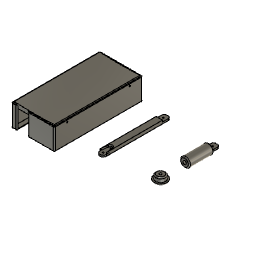
WP_Switch v2 (Autodesk Fusion 360 design; units mm, degrees)
Autodesk Fusion 360 part; units mm, degrees
sketch "Skizze1" plane through (0, 0, 0) normal (0, 1, 0) x (1, 0, 0)
  line L0 (18.75, -0.5552) -> (18.75, 3.444)
  line L1 (18.75, 3.444) -> (-18.75, 3.444)
  line L2 (-18.75, 3.444) -> (-18.75, -0.556)
  arc A0 (18.75, -0.5552) -> (-18.75, -0.556) centre (0.0063, -299.9691) ccw
  dimension "d1" = 600
  dimension "d2" = 37.5
  dimension "d3" = 18.75
  dimension "d4" = 4
  constraint vertical L0
  constraint horizontal L1
  constraint vertical L2
  measures "d1" diameter of A0
  measures "d2" distance of L2.end L0.start
  measures "d3" horizontal distance of origin L2.end
  measures "d4" distance of L2.end L1.end
extrude "Extrusion2" add sketch "Skizze1" along normal blind 80 makes body 1
sketch "Skizze2" plane through (0, 0, -3.444) normal (0, 0, -1) x (1, 0, 0)
  line L0 (18.75, 0) -> (-18.75, 0)
  line L1 (-18.75, 0) -> (-18.75, -80)
  line L2 (-18.75, -80) -> (18.75, -80)
  line L3 (18.75, -80) -> (18.75, 0)
  line L4 (-18.75, 0) -> (18.75, -80) construction
  line L5 (18.75, 0) -> (-18.75, -80) construction
  line L6 (19, 0.25) -> (-19, 0.25)
  line L7 (-19, 0.25) -> (-19, -80.25)
  line L8 (-19, -80.25) -> (19, -80.25)
  line L9 (19, -80.25) -> (19, 0.25)
  line L10 (19, 0.25) -> (-19, -80.25) construction
  line L11 (-19, 0.25) -> (19, -80.25) construction
  line L12 (-20, -81.25) -> (20, -81.25)
  line L13 (20, -81.25) -> (20, 1.25)
  line L14 (20, 1.25) -> (-20, 1.25)
  line L15 (-20, 1.25) -> (-20, -81.25)
  point P0 (0, -40)
  dimension "d9" = 38
  dimension "d10" = 80.5
  dimension "d11" = 1
  constraint coincident L0.end L1.start
  constraint coincident L2.end L3.start
  constraint coincident L0.start L3.end
  constraint coincident L1.end L2.start
  constraint horizontal L6
  constraint perpendicular L6 L7
  constraint parallel L6 L8
  constraint parallel L7 L9
  constraint coincident L10 P0
  constraint coincident L11 P0
  constraint midpoint L5 P0
  measures "d9" distance of L7.end L8.end
  measures "d10" distance of L6.end L7.end
extrude "Extrusion3" add sketch "Skizze2" along normal blind 16 and the other way blind 3 separate body contours L12 L13 L14 L15 makes body 2
sketch "Skizze3" plane through (0, 0, -3.444) normal (0, 0, -1) x (1, 0, 0)
  line L0 (18.75, 0) -> (-18.75, 0)
  line L1 (-18.75, 0) -> (-18.75, -80)
  line L2 (-18.75, -80) -> (18.75, -80)
  line L3 (18.75, -80) -> (18.75, 0)
  line L4 (-1, -3.1253) -> (6, -3.1253)
  line L5 (6, -3.1253) -> (6, -8.3753)
  line L6 (6, -8.3753) -> (-1, -8.3753)
  line L7 (-1, -8.3753) -> (-1, -3.1253)
  line L8 (-1, -28.3753) -> (6, -28.3753)
  line L9 (6, -28.3753) -> (6, -33.6253)
  line L10 (6, -33.6253) -> (-1, -33.6253)
  line L11 (-1, -33.6253) -> (-1, -28.3753)
  line L12 (-1, -8.3753) -> (-1, -28.3753) construction
  line L13 (-18.75, 0) -> (18.75, -80) construction
  line L14 (18.75, 0) -> (-18.75, -80) construction
  line L15 (-16.9509, -3.8381) -> (16.9509, -3.8381)
  line L16 (16.9509, -3.8381) -> (16.9509, -33.6785)
  line L17 (16.9509, -33.6785) -> (-16.9509, -33.6785)
  line L18 (-16.9509, -33.6785) -> (-16.9509, -3.8381)
  dimension "d16" = 7
  dimension "d17" = 5.25
  dimension "d18" = 7
  dimension "d19" = 5.25
  dimension "d20" = 20
  dimension "d23" = 1
  constraint horizontal L4
  constraint vertical L5
  constraint horizontal L6
  constraint vertical L7
  constraint horizontal L8
  constraint vertical L9
  constraint horizontal L10
  constraint vertical L11
  constraint perpendicular L8 L12
  constraint coincident L0.end L1.start
  constraint coincident L2.end L3.start
  constraint coincident L0.start L3.end
  constraint coincident L1.end L2.start
  constraint horizontal L15
  constraint vertical L16
  constraint horizontal L17
  constraint vertical L18
  constraint coincident L13 L15.start
  constraint coincident L14 L15.end
  measures "d16" distance of L4.start L4.end
  measures "d17" distance of L4.start L6.end
  measures "d18" distance of L8.start L8.end
  measures "d19" distance of L8.end L9.end
  measures "d20" distance of L6.end L8.start
  measures "d23" horizontal distance of origin L4.start
extrude "Extrusion4" add sketch "Skizze3" along normal blind 1.5 separate body contours L5 L6 L7 L15 L16 L17 L18 makes body 3
extrude "Extrusion5" add sketch "Skizze3" along normal blind 9 contours L4 L5 L7 L15 | L5 L6 L7 L15 | L8 L9 L10 L11 bodies 1 3
ref_plane "Arbeitsebene1" through (0, 40, -3.444) normal (0, 0, -1) x (-1, 0, 0)
split "Teilen1" by plane through (0, 40, -3.444) normal (0, 0, -1) bodies 1 makes body 4 at (-11.6339, 21.9639, -4.944)
sketch "Skizze5" plane through (0, 0, -19.444) normal (0, 0, -1) x (1, 0, 0)
  line L0 (19, 0.25) -> (19, -80.25)
  line L1 (19, -80.25) -> (-19, -80.25)
  line L2 (-19, -80.25) -> (-19, 0.25)
  line L3 (-19, 0.25) -> (19, 0.25)
  line L4 (-20, 1.25) -> (-20, -81.25)
  line L5 (-20, -81.25) -> (20, -81.25)
  line L6 (20, -81.25) -> (20, 1.25)
  line L7 (20, 1.25) -> (-20, 1.25)
  line L8 (20, -81.25) -> (-20, -81.25)
  line L9 (-20, -81.25) -> (-20, 1.25)
  line L10 (-20, 1.25) -> (20, 1.25)
  line L11 (20, 1.25) -> (20, -81.25)
  constraint horizontal L8
  constraint vertical L9
  constraint horizontal L10
  constraint vertical L11
  constraint coincident L4.start L7.end
  constraint coincident L5.end L6.start
extrude "Extrusion8" add sketch "Skizze5" along normal blind 1.5 contours L0 L1 L2 L3 | L4 L5 L6 L7 L8 L9 L10 L11 bodies 2
move_body "Verschieben2" bodies 4 to x (1, 0, 0) y (0, 1, 0) z (0, 0, 1) at (2, 0, 0)
sketch "Skizze7" plane through (0, 0, -20.944) normal (0, 0, -1) x (1, 0, 0)
  line L0 (20, 1.25) -> (-20, 1.25)
  line L1 (-20, 1.25) -> (-20, -81.25)
  line L2 (-20, -81.25) -> (20, -81.25)
  line L3 (20, -81.25) -> (20, 1.25)
  line L4 (-15, 5.4864) -> (-5, 5.4864)
  line L5 (-5, 5.4864) -> (-5, -16.3923)
  line L6 (-5, -16.3923) -> (-15, -16.3923)
  line L7 (-15, -16.3923) -> (-15, 5.4864)
  dimension "d48" = 5
  dimension "d49" = 10
  constraint horizontal L4
  constraint vertical L5
  constraint horizontal L6
  constraint vertical L7
  measures "d48" horizontal distance of origin L4.end
  measures "d49" distance of L4.start L4.end
extrude "Extrusion9" cut sketch "Skizze7" against normal blind 40 contours L0 L5 L6 L7 | L0 L4 L5 L7 bodies 2
sketch "Skizze8" plane through (8, 0, 0) normal (1, 0, 0) x (0, 1, 0)
  line L0 (33.6253, -4.944) -> (28.3753, -4.944)
  line L1 (28.3753, -4.944) -> (28.3753, -12.444)
  line L2 (28.3753, -12.444) -> (33.6253, -12.444)
  line L3 (33.6253, -12.444) -> (33.6253, -4.944)
  point P0 (30.0753, -9.244)
  point P1 (6.5753, -9.244)
  point P2 (8.3753, -12.444)
  point P3 (8.3753, -4.944)
  dimension "d53" = 23.5
  dimension "d54" = 1.8
  dimension "d55" = 4.3
  measures "d53" distance of P0 P1
  measures "d54" horizontal distance of P1 P2
  measures "d55" vertical distance of P1 P3
fillet "Abrundung2" radius 2 2 edges at (1, 6.1067, -4.944) (1, 31.0003, -4.944) on bodies 4
fillet "Abrundung2" radius 1 8 edges at (4.5, 28.3753, -12.444) (8, 31.0003, -12.444) (4.5, 33.6253, -12.444) (1, 31.0003, -12.444) (8, 5.7503, -12.444) (4.5, 3.1253, -12.444) (1, 5.7503, -12.444) (4.5, 8.3753, -12.444) on bodies 4
hole "Bohrung2" at (8, 30.0753, -9.244) at (8, 6.5753, -9.244) direction (-1, 0, 0) diameter 1.8 depth 9 tip angle 118 bodies 4
sketch "Skizze9" plane through (20, 0, 0) normal (1, 0, 0) x (0, 1, 0)
  line L0 (-1.25, -0.444) -> (-1.25, -20.944)
  line L1 (-1.25, -20.944) -> (81.25, -20.944)
  line L2 (81.25, -20.944) -> (81.25, -0.444)
  line L3 (81.25, -0.444) -> (-1.25, -0.444)
  line L4 (81.25, -2.244) -> (-1.25, -2.244) construction
  point P0 (69.25, -2.244)
  point P1 (10.75, -2.244)
  dimension "d64" = 1.8
  dimension "d65" = 12
  dimension "d66" = 12
  constraint coincident L2 L4.start
  constraint coincident L0 L4.end
  constraint perpendicular L0 L4
  constraint coincident L4 P0
  constraint coincident L4 P1
  measures "d64" distance of L2.end L4.start
  measures "d65" distance of L4.start P0
  measures "d66" distance of L4.end P1
ref_plane "Arbeitsebene2" through (0, 25, 0) normal (0, 1, 0) x (0, 0, 1)
sketch "Skizze10" plane through (-20, 0, 0) normal (-1, 0, 0) x (0, -1, 0)
  line L0 (-81.25, -0.444) -> (-81.25, -20.944)
  line L1 (-81.25, -20.944) -> (1.25, -20.944)
  line L2 (1.25, -20.944) -> (1.25, -0.444)
  line L3 (1.25, -0.444) -> (-81.25, -0.444)
  line L4 (1.25, -2.244) -> (-81.25, -2.244) construction
  point P0 (-10.75, -2.244)
  point P1 (-69.25, -2.244)
  dimension "d67" = 1.8
  dimension "d68" = 12
  dimension "d69" = 12
  constraint coincident L2 L4.start
  constraint coincident L0 L4.end
  constraint perpendicular L0 L4
  constraint coincident L4 P0
  constraint coincident L4 P1
  measures "d67" distance of L2.end L4.start
  measures "d68" distance of L4.start P0
  measures "d69" distance of L4.end P1
hole "Bohrung3" at (-20, 10.75, -2.244) at (-20, 69.25, -2.244) direction (1, 0, 0) diameter 1.3 depth 9 tip angle 118 bodies 1 2
hole "Bohrung4" at (20, 69.25, -2.244) at (20, 10.75, -2.244) direction (-1, 0, 0) diameter 1.3 depth 9 tip angle 118 bodies 1 2
sketch "Skizze11" plane through (0, 0, 0) normal (0, 0, 1) x (1, 0, 0)
  line L0 (65.0969, 6.2494) -> (63.0969, 6.2494) construction
  line L1 (65.0969, 6.2494) -> (67.0969, 6.2494) construction
  line L2 (65.0969, -0.7506) -> (62.0969, -0.7538) construction
  line L3 (65.0969, -0.7506) -> (68.0969, -0.7473) construction
  line L4 (63.0969, 6.2494) -> (62.2157, 0.0851)
  line L5 (67.0969, 6.2494) -> (68.0969, -0.7473)
  arc A0 (62.2157, 0.0851) -> (68.0969, -0.7473) centre (65.0969, -0.7506) ccw
  line L6 (65.0969, 6.2494) -> (65.0969, -0.7506) construction
  line L7 (62.0969, -0.7538) -> (68.0969, -0.7538) construction
  line L8 (68.0969, -0.7538) -> (68.0969, 59.2462)
  line L9 (68.0969, 59.2462) -> (62.0969, 59.2462)
  line L10 (62.0969, 59.2462) -> (62.0969, -0.7538)
  arc A1 (67.0969, 6.2494) -> (63.0969, 6.2494) centre (65.0969, 6.2494) ccw
  line L11 (62.0969, 51.7289) -> (68.0969, 51.7289)
  line L12 (62.0969, 59.2462) -> (68.0969, 51.7289) construction
  line L13 (68.0969, 59.2462) -> (62.0969, 51.7289) construction
  dimension "d78" = 6
  dimension "d79" = 4
  dimension "d80" = 7
  dimension "d83" = 60
  constraint coincident L0.start L1.start
  constraint coincident L2.start L3.start
  constraint coincident L2.end A0
  constraint parallel L2 L3
  constraint vertical L6
  constraint horizontal L7
  constraint vertical L8
  constraint horizontal L9
  constraint vertical L10
  constraint coincident L10 L11.start
  constraint coincident L8 L11.end
  constraint perpendicular L8 L11
  measures "d78" diameter of A0
  measures "d79" diameter of A1
  measures "d80" distance of L2.start L0.start
  measures "d83" distance of L2.end L9.end
extrude "Extrusion10" add sketch "Skizze11" along normal blind 3 separate body contours L4 L5 A0 L8 L10 A1 L11 makes body 5
extrude "Extrusion11" add sketch "Skizze11" along normal blind 1.5 contours L4 L5 A0 L8 A1 | L8 L9 L10 L11 bodies 5
sketch "Skizze12" plane through (0, 0, 1.5) normal (0, 0, 1) x (-1, 0, 0)
  line L0 (-68.0969, 0.7473) -> (-67.0969, -6.2494)
  arc A0 (-67.0969, -6.2494) -> (-63.0969, -6.2494) centre (-65.0969, -6.2494) ccw
  line L1 (-63.0969, -6.2494) -> (-62.2157, -0.0851)
  arc A1 (-62.2157, -0.0851) -> (-62.0969, 0.7538) centre (-65.0969, 0.7506) ccw
  arc A2 (-62.0969, 0.7538) -> (-68.0969, 0.7538) centre (-65.0969, 0.7506) ccw
  point P0 (-65.0969, -6.2494)
  point P1 (-65.0969, 0.7506)
  point P2 (-65.0947, -55.4807)
  constraint coincident P0 A0.centre
  constraint coincident P1 A1.centre
hole "Bohrung5" at (65.0969, -0.7506, 1.5) at (65.0969, 6.2494, 1.5) at (65.0947, 55.4807, 1.5) direction (0, 0, -1) diameter 1.3 depth 9 tip angle 118 bodies 5
fillet "Abrundung3" radius 2 2 edges at (62.0969, 59.2462, 0.75) (68.0969, 59.2462, 0.75) on bodies 5
copy_body "Körper kopieren/einfügen1" bodies 5 makes body 6
move_body "Verschieben3" bodies 6 to x (1, 0, 0) y (0, 1, 0) z (0, 0, 1) at (46, 0, 0)
sketch "Skizze13" plane through (0, 0, 3) normal (0, 0, 1) x (-1, 0, 0)
  line L0 (-113.0969, -6.2494) -> (-114.0969, 0.7473)
  line L1 (-114.0969, 0.7473) -> (-114.0969, -51.7289)
  line L2 (-114.0969, -51.7289) -> (-108.0969, -51.7289)
  line L3 (-108.0969, -51.7289) -> (-108.0969, 0.7538)
  arc A0 (-108.2157, -0.0851) -> (-108.0969, 0.7538) centre (-111.0969, 0.7506) ccw
  line L4 (-108.2157, -0.0851) -> (-109.0969, -6.2494)
  arc A1 (-113.0969, -6.2494) -> (-109.0969, -6.2494) centre (-111.0969, -6.2494) ccw
  line L5 (-106.8497, -29.2462) -> (-116.469, -29.2462)
  line L6 (-116.469, -29.2462) -> (-116.469, 8.7404)
  line L7 (-116.469, 8.7404) -> (-106.8497, 8.7404)
  line L8 (-106.8497, 8.7404) -> (-106.8497, -29.2462)
  point P0 (-112.0969, -59.2462)
  dimension "d93" = 30
  constraint horizontal L5
  constraint vertical L6
  constraint horizontal L7
  constraint vertical L8
  measures "d93" vertical distance of L5.end P0
extrude "Extrusion12" cut sketch "Skizze13" against normal blind 5 contours L0 L1 L3 A0 L4 A1 L5 | L0 L1 L3 A0 L4 A1 L5 L6 L7 L8 bodies 6
sketch "Skizze14" plane through (0, 29.2462, 0) normal (0, -1, 0) x (1, 0, 0)
  line L0 (114.0969, 0) -> (114.0969, 3)
  line L1 (114.0969, 3) -> (108.0969, 3)
  line L2 (108.0969, 3) -> (108.0969, 0)
  line L3 (108.0969, 0) -> (114.0969, 0)
  circle A0 centre (111.0969, 1.4239) radius 4.5
  dimension "d96" = 9
  measures "d96" diameter of A0
extrude "Extrusion13" add sketch "Skizze14" against normal blind 22 contours L0 L1 L2 L3 | A0 bodies 6
sketch "Skizze15" plane through (0, 0, 0) normal (0, 0, 1) x (1, 0, 0)
  circle A0 centre (111.556, 6.4045) radius 4.5
  circle A1 centre (111.556, 6.4045) radius 6
  dimension "d99" = 9
  dimension "d100" = 12
  constraint concentric A0 A1
  measures "d99" diameter of A0
  measures "d100" diameter of A1
extrude "Extrusion14" add sketch "Skizze15" along normal blind 4 separate body contours A0 makes body 7
extrude "Extrusion15" add sketch "Skizze15" against normal blind 2 contours A0 | A1 bodies 7
fillet "Abrundung4" radius 1 1 edges at (106.9014, 29.2462, -0.2034) on bodies 6 7
fillet "Abrundung4" radius 2 1 edges at (105.9621, 8.5742, -2) on bodies 6 7
fillet "Abrundung4" radius 1 1 edges at (107.3606, 4.7772, 4) on bodies 6 7
sketch "Skizze16" plane through (0, 29.2462, 0) normal (0, -1, 0) x (1, 0, 0)
  circle A0 centre (111.0969, 1.4239) radius 3.5
  point P0 (111.0969, 1.4239)
  constraint coincident P0 A0.centre
sketch "Skizze17" plane through (0, 0, 4) normal (0, 0, 1) x (-1, 0, 0)
  circle A0 centre (-111.556, -6.4045) radius 3.5
  point P0 (-111.556, -6.4045)
  constraint coincident P0 A0.centre
hole "Bohrung6" at (111.0969, 29.2462, 1.4239) direction (0, 1, 0) diameter 3.2 depth 10 tip angle 118 bodies 6
hole "Bohrung7" at (111.556, 6.4045, 4) direction (0, 0, -1) diameter 2.2 depth 4 tip angle 118 bodies 7
sketch "Skizze18" plane through (0, 81.25, 0) normal (0, 1, 0) x (-1, 0, 0)
  line L0 (-20, -0.444) -> (-20, -20.944)
  line L1 (-20, -20.944) -> (20, -20.944)
  line L2 (20, -20.944) -> (20, -0.444)
  line L3 (20, -0.444) -> (-20, -0.444)
  line L4 (10.9992, -15.2307) -> (18.1992, -15.2307)
  line L5 (18.1992, -15.2307) -> (18.1992, -19.4307)
  line L6 (18.1992, -19.4307) -> (10.9992, -19.4307)
  line L7 (10.9992, -19.4307) -> (10.9992, -15.2307)
  line L8 (10.9992, -15.2307) -> (18.1992, -19.4307) construction
  line L9 (18.1992, -15.2307) -> (10.9992, -19.4307) construction
  point P0 (14.5992, -17.3307)
  dimension "d117" = 7.2
  dimension "d118" = 4.2
  constraint horizontal L4
  constraint perpendicular L4 L5
  constraint parallel L4 L6
  constraint parallel L5 L7
  constraint coincident L8 P0
  constraint coincident L9 P0
  measures "d117" distance of L5.end L6.end
  measures "d118" distance of L4.end L5.end
extrude "Extrusion16" cut sketch "Skizze18" against normal blind 3 contours L4 L5 L6 L7 bodies 2
sketch "Skizze19" plane through (0, 0, -20.944) normal (0, 0, -1) x (1, 0, 0)
  line L0 (-19, -39.75) -> (19, -39.75) construction
  circle A0 centre (-4, -39.75) radius 1.6
  circle A1 centre (4, -39.75) radius 1.6
  line L1 (-5, 1.25) -> (-5, -16.3923)
  line L2 (-5, -16.3923) -> (-15, -16.3923)
  line L3 (-15, -16.3923) -> (-15, 1.25)
  line L4 (-15, 1.25) -> (-20, 1.25)
  line L5 (-20, 1.25) -> (-20, -81.25)
  line L6 (-20, -81.25) -> (20, -81.25)
  line L7 (20, -81.25) -> (20, 1.25)
  line L8 (20, 1.25) -> (-5, 1.25)
  dimension "d126" = 3.2
  dimension "d127" = 3.2
  dimension "d128" = 15
  dimension "d129" = 15
  constraint coincident L0 A0.centre
  constraint coincident L0 A1.centre
  measures "d126" diameter of A0
  measures "d127" diameter of A1
  measures "d128" distance of L0.start A0.centre
  measures "d129" distance of L0.end A1.centre
extrude "Extrusion17" cut sketch "Skizze19" against normal blind 2 contours A0 | A1 bodies 2
sketch "Skizze20" plane through (0, 0, -19.444) normal (0, 0, 1) x (-1, 0, 0)
  circle A0 centre (-4, -39.75) radius 1.6
  circle A1 centre (4, -39.75) radius 1.6
  line L0 (19, -80.25) -> (19, 0.25)
  line L1 (5, 0.25) -> (-19, 0.25)
  line L2 (15, 0.25) -> (15, -16.3923)
  line L3 (15, -16.3923) -> (5, -16.3923)
  line L4 (5, -16.3923) -> (5, 0.25)
  line L5 (-19, 0.25) -> (-19, -80.25)
  line L6 (-19, -80.25) -> (19, -80.25)
  circle A2 centre (4, -39.75) radius 2.5
  circle A3 centre (-4, -39.75) radius 2.5
  circle A4 centre (4, -39.75) radius 2
  circle A5 centre (-4, -39.75) radius 2
  line L7 (19, 0.25) -> (15, 0.25)
  dimension "d132" = 5
  dimension "d133" = 5
  dimension "d134" = 4
  dimension "d135" = 4
  constraint concentric A1 A2
  constraint concentric A0 A3
  constraint concentric A2 A4
  constraint concentric A3 A5
  measures "d132" diameter of A2
  measures "d133" diameter of A3
  measures "d134" diameter of A4
  measures "d135" diameter of A5
extrude "Extrusion18" add sketch "Skizze20" along normal blind 1 contours A4 | A5 bodies 2
extrude "Extrusion19" add sketch "Skizze20" along normal blind 2 contours A2 | A3 bodies 2
fillet "Abrundung6" radius 1 14 edges at (-20, 40, -20.944) (-17.5, -1.25, -20.944) (-15, -1.25, -10.694) (-15, 7.5711, -20.944) (-10, 16.3923, -20.944) (-5, 7.5711, -20.944) (7.5, -1.25, -20.944) (20, -1.25, -10.694) (20, 40, -20.944) (20, 81.25, -10.694) (0, 81.25, -20.944) (-20, 81.25, -10.694) (-20, -1.25, -10.694) (-5, -1.25, -10.694) on bodies 2
fillet "Abrundung6" radius 0.5 4 edges at (-10.9992, 81.25, -17.3307) (-14.5992, 81.25, -19.4307) (-18.1992, 81.25, -17.3307) (-14.5992, 81.25, -15.2307) on bodies 2
equation "d3 = d2 / 2"
equation "d18 = d16"
equation "d19 = d17"
equation "d66 = d65"
